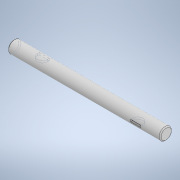
# Autodesk Inventor part: Mainpulo
Saved by Autodesk Inventor 2021 (Build 250183000, 183)
## iProperties
Created: 2022-02-22
Part Number: Mainpulo
Material: Genérico
Document SubType Name: Modeling
Designer: aluno
Density: 1 g/cm^3
Appearance: Padrão
Author: aluno
Autodesk Inventor part; units mm, degrees
ref_plane "YZ Plane" through (0, 0, 0) normal (1, 0, 0) x (0, 1, 0)
ref_plane "XZ Plane" through (0, 0, 0) normal (0, 1, 0) x (-1, 0, 0)
ref_plane "XY Plane" through (0, 0, 0) normal (0, 0, 1) x (1, 0, 0)
sketch "Esboço1" plane through (0, 0, 0) normal (0, 0, 1) x (1, 0, 0)
  line L0 (0, 0) -> (75, 0)
  line L1 (75, 0) -> (75, 3)
  line L2 (75, 3) -> (0, 3)
  line L3 (0, 3) -> (0, 0)
  dimension "d0" = 75
  dimension "d1" = 3
  constraints: 8 end point, 2 parallel, 1 horizontal, 1 perpendicular
  measures "d0" distance of L2.end L1.end
  measures "d1" distance of L1.end L0.end
revolve "Revolução1" add sketch "Esboço1" angle 360 about axis through (0, 0, 0) along (1, 0, 0)
sketch "Esboço2" plane through (0, 0, 0) normal (0, 1, 0) x (-1, 0, 0)
  point P0 (0, 0)
chamfer "Chanfro1" distance 0.5 angle 45 2 edges at (0, -3, 0) (75, -3, 0)
sketch "Esboço3" plane through (0, 0, 0) normal (0, 1, 0) x (-1, 0, 0)
  line L0 (0, 2.5) -> (0, -2.5) projected
  line L1 (-75, 2.5) -> (-74.5, 3) projected
  line L2 (-74.5, 3) -> (-0.5, 3) projected
  line L3 (-0.5, 3) -> (0, 2.5) projected
  line L4 (0, 2.5) -> (0, -2.5) projected
  line L5 (0, -2.5) -> (-0.5, -3) projected
  line L6 (-0.5, -3) -> (-74.5, -3) projected
  line L7 (-74.5, -3) -> (-75, -2.5) projected
  line L8 (-75, -2.5) -> (-75, 2.5) projected
  line L9 (-0.5, -3) -> (-74.5, -3) projected
  line L10 (-14.5, -2) -> (-14.5, -3)
  line L11 (-9.5, -3) -> (-9.5, -2)
  arc A0 (-9.5, -2) -> (-14.5, -2) centre (-12, -2) ccw
  arc A1 (-14.2913, -3) -> (-9.7087, -3) centre (-12, -2) ccw
  line L12 (-14.5, -3) -> (-14.2913, -3)
  line L13 (-9.7087, -3) -> (-9.5, -3)
  line L14 (-65.5, 2) -> (-65.5, 3)
  line L15 (-60.5, 3) -> (-60.5, 2)
  arc A2 (-60.7087, 3) -> (-65.2913, 3) centre (-63, 2) ccw
  arc A3 (-65.5, 2) -> (-60.5, 2) centre (-63, 2) ccw
  line L16 (-65.5, 3) -> (-65.2913, 3)
  line L17 (-60.7087, 3) -> (-60.5, 3)
  point P0 (0, 0)
  point P1 (-14.2913, -3)
  point P2 (-9.7087, -3)
  point P3 (-9.7087, -3)
  point P4 (-14.2913, -3)
  dimension "d10" = 12
  dimension "d12" = 12
  constraints: 16 end point, 8 point on circle, 4 centre point, 2 parallel, 2 point on line
  measures "d10" distance from line of L8 A2.centre
  measures "d12" distance from line of L0 A0.centre
extrude "Extrusão1" cut sketch "Esboço3" against normal mid plane 1 contours L15 A3 L14 L2 | L6 L10 A0 L11 | L2 A2 | A1 L6
